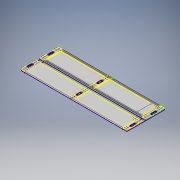
# Autodesk Inventor part: Fixture Base
Saved by Autodesk Inventor 2018 (Build 220112000, 112)
## iProperties
Created: 2016-04-07
Part Number: Fixture Base
Material: Generic
Document SubType Name: Modeling
Designer: Sam Clay
Density: 1 g/cm^3
Appearance: Default
Author: Sam Clay
Autodesk Inventor part; units mm, degrees
ref_plane "YZ Plane" through (0, 0, 0) normal (1, 0, 0) x (0, 1, 0)
ref_plane "XZ Plane" through (0, 0, 0) normal (0, 1, 0) x (-1, 0, 0)
ref_plane "XY Plane" through (0, 0, 0) normal (0, 0, 1) x (1, 0, 0)
sketch "Base Sketch" plane through (0, 0, 0) normal (0, 1, 0) x (-1, 0, 0)
  line L0 (0, 0) -> (1320.8, 0)
  line L1 (1320.8, 0) -> (1320.8, 254)
  line L2 (1320.8, 508) -> (0, 508)
  line L3 (0, 508) -> (0, 304.8)
  line L4 (0, 508) -> (-50.8, 508)
  line L5 (-50.8, 508) -> (-50.8, 304.8)
  line L6 (-50.8, 0) -> (0, 0)
  line L7 (0, 0) -> (0, 254)
  line L8 (1320.8, 508) -> (1371.6, 508)
  line L9 (1371.6, 508) -> (1371.6, 304.8)
  line L10 (1371.6, 0) -> (1320.8, 0)
  line L11 (1320.8, 0) -> (1320.8, 254)
  line L12 (1320.8, 254) -> (1320.8, 304.8)
  line L13 (1371.6, 254) -> (1371.6, 0)
  line L14 (0, 254) -> (0, 254)
  line L15 (-50.8, 254) -> (-50.8, 0)
  line L16 (1371.6, 254) -> (1320.8, 254)
  line L17 (1371.6, 304.8) -> (1320.8, 304.8)
  line L18 (1371.6, 304.8) -> (1371.6, 254)
  line L19 (1371.6, 254) -> (1371.6, 254)
  line L20 (1320.8, 254) -> (1320.8, 304.8)
  line L21 (1320.8, 304.8) -> (1320.8, 508)
  line L22 (0, 304.8) -> (0, 254)
  line L23 (0, 254) -> (0, 304.8)
  line L24 (-50.8, 254) -> (-50.8, 254)
  line L25 (-50.8, 304.8) -> (-50.8, 254)
  line L26 (1320.8, 254) -> (0, 254)
  line L27 (1320.8, 304.8) -> (0, 304.8)
  line L28 (0, 304.8) -> (-50.8, 304.8)
  line L29 (0, 254) -> (-50.8, 254)
  line L30 (0, 304.8) -> (0, 508)
  line L31 (0, 254) -> (0, 0)
  line L32 (1320.8, 254) -> (1320.8, 304.8)
  line L33 (1320.8, 304.8) -> (1320.8, 508)
  line L34 (1308.1, 0) -> (1308.1, 254)
  line L35 (12.7, 0) -> (12.7, 254)
  line L36 (1308.1, 304.8) -> (1308.1, 508) construction
  line L37 (12.7, 304.8) -> (12.7, 508) construction
  line L38 (1289.05, 323.85) -> (31.75, 323.85) construction
  line L39 (31.75, 323.85) -> (31.75, 488.95) construction
  line L40 (31.75, 488.95) -> (1289.05, 488.95) construction
  line L41 (1289.05, 488.95) -> (1289.05, 323.85) construction
  line L42 (660.4, 0) -> (660.4, 254)
  line L43 (660.4, 304.8) -> (660.4, 508)
  line L44 (711.2, 0) -> (711.2, 254)
  line L45 (711.2, 304.8) -> (711.2, 508)
  line L46 (647.7, 0) -> (647.7, 254)
  line L47 (647.7, 304.8) -> (647.7, 508) construction
  line L48 (628.65, 323.85) -> (628.65, 488.95) construction
  dimension "d89" = 17.78
  dimension "d0" = 1320.8
  dimension "d87" = 50.8
  dimension "d88" = 50.8
  dimension "d165" = 254
  dimension "d166" = 50.8
  dimension "d167" = 203.2
  dimension "d172" = 12.7
  dimension "d173" = 12.7
  dimension "d213" = 12.7
  dimension "d214" = 12.7
  dimension "d215" = 19.05
  dimension "d216" = 19.05
  dimension "d217" = 19.05
  dimension "d218" = 19.05
  dimension "d221" = 660.4
  dimension "d222" = 50.8
  dimension "d230" = 12.7
  dimension "d231" = 12.7
  dimension "d232" = 19.05
  constraints: 98 end point, 45 parallel, 40 perpendicular, 28 point on line, 14 coincident, 4 horizontal, 4 midpoint
  measures "d0" distance of L2.end L2.start
  measures "d87" distance of L6.end L6.start
  measures "d88" distance of L10.start L10.end
  measures "d165" distance between parallel lines of L16 L0
  measures "d166" distance between parallel lines of L16 L17
  measures "d167" distance between parallel lines of L2 L17
  measures "d172" distance between parallel lines of L34 L1
  measures "d173" distance between parallel lines of L31 L35
  measures "d213" distance between parallel lines of L33 L36
  measures "d214" distance between parallel lines of L3 L37
  measures "d215" distance between parallel lines of L38 L27
  measures "d216" distance between parallel lines of L36 L41
  measures "d217" distance between parallel lines of L37 L39
  measures "d218" distance between parallel lines of L2 L40
  measures "d221" distance between parallel lines of L42 L31
  measures "d222" distance between parallel lines of L44 L42
  measures "d230" distance between parallel lines of L46 L42
  measures "d231" distance between parallel lines of L47 L43
  measures "d232" distance between parallel lines of L48 L47
extrude "Lower Level" add sketch "Base Sketch" along normal blind 17.78 contours L6 L15 L29 L7 | L28 L5 L4 L3 | L21 L8 L9 L17 | L1 L16 L13 L10
extrude "Base" add sketch "Base Sketch" along normal blind 19.05 contours L7 L26 L35 L0 | L35 L26 L46 L0 | L46 L26 L42 L0 | L3 L2 L43 L27 | L42 L26 L44 L0 | L43 L2 L45 L27 | L44 L26 L34 L0 | L45 L2 L21 L27 | L34 L26 L1 L0
sketch "Tracks Sketch" plane through (0, 19.05, 0) normal (0, 1, 0) x (1, 0, 0)
  line L0 (-1320.8, 0) -> (-1320.8, -254) projected
  line L1 (0, -254) -> (0, 0) projected
  line L2 (-1320.8, -22.987) -> (0, -22.987)
  line L3 (-1320.8, -3.175) -> (0, -3.175)
  line L4 (-1320.8, -231.013) -> (0, -231.013)
  line L5 (-1320.8, -250.825) -> (0, -250.825)
  line L6 (-88.9, -40.767) -> (-1320.8, -40.767)
  line L7 (-1320.8, -40.767) -> (-1320.8, -231.013)
  line L8 (-88.9, -231.013) -> (-88.9, -40.767)
  circle A0 centre (-92.71, -44.577) radius 8.89
  line L9 (-1371.6, 0) -> (-1371.6, -254) projected
  line L10 (50.8, -508) -> (50.8, -304.8) projected
  line L11 (-1371.6, -508) -> (50.8, -508) projected
  line L12 (50.8, -304.8) -> (-1371.6, -304.8) projected
  line L13 (-1371.6, -254) -> (50.8, -254) projected
  line L14 (50.8, 0) -> (-1371.6, 0) projected
  line L15 (-1371.6, -304.8) -> (-1371.6, -508) projected
  line L16 (50.8, -254) -> (50.8, 0) projected
  point P0 (-660.4, -254)
  point P1 (-1320.8, -223.393)
  point P2 (-1422.4, -254)
  dimension "d170" = 19.812
  dimension "d171" = 19.812
  dimension "d174" = 88.9
  dimension "d175" = 17.78
  dimension "d178" = 17.78
  dimension "d179" = 5.08
  dimension "d180" = 5.08
  dimension "d219" = 3.175
  dimension "d220" = 3.175
  constraints: 14 end point, 6 point on line, 5 perpendicular, 1 centre point, 1 horizontal, 1 parallel, 6 other
  measures "d170" distance between parallel lines of L5 L4
  measures "d171" distance between parallel lines of L2 L3
  measures "d174" distance between parallel lines of L1 L8
  measures "d175" distance between parallel lines of L2 L6
  measures "d178" diameter of A0
  measures "d179" distance edge to line of A0 L6
  measures "d180" distance edge to line of A0 L8
  measures "d219" distance between parallel lines of L14 L3
  measures "d220" distance between parallel lines of L13 L5
extrude "Pocket side" cut sketch "Tracks Sketch" against normal blind 3.175 contours L6 A0 L8 L4 L0 | A0 L8 L6 | L6 L8 A0
extrude "Tracks" cut sketch "Tracks Sketch" against normal blind 11.43 contours L3 L1 L2 L0 | L4 L1 L5 L0
sketch "Handle Sketch" plane through (0, 17.78, 0) normal (0, 1, 0) x (1, 0, 0)
  line L0 (-1371.6, -254) -> (-1320.8, -254) projected
  line L1 (-1320.8, -40.767) -> (-1320.8, -22.987) projected
  line L2 (-1320.8, -22.987) -> (-1320.8, -3.175) projected
  line L3 (-1320.8, -250.825) -> (-1320.8, -40.767) projected
  line L4 (-1320.8, -254) -> (-1320.8, -250.825) projected
  line L5 (-1320.8, -3.175) -> (-1320.8, 0) projected
  line L6 (-1320.8, 0) -> (-1371.6, 0) projected
  line L7 (-1371.6, 0) -> (-1371.6, -254) projected
  line L8 (50.8, 0) -> (0, 0) projected
  line L9 (0, 0) -> (0, -3.175) projected
  line L10 (0, -3.175) -> (0, -22.987) projected
  line L11 (0, -22.987) -> (0, -231.013) projected
  line L12 (0, -231.013) -> (0, -250.825) projected
  line L13 (0, -250.825) -> (0, -254) projected
  line L14 (0, -254) -> (50.8, -254) projected
  line L15 (50.8, -254) -> (50.8, 0) projected
  line L16 (0, -508) -> (50.8, -508) projected
  line L17 (50.8, -508) -> (50.8, -304.8) projected
  line L18 (50.8, -304.8) -> (0, -304.8) projected
  line L19 (0, -304.8) -> (0, -508) projected
  line L20 (-1320.8, -508) -> (-1320.8, -304.8) projected
  line L21 (-1320.8, -304.8) -> (-1371.6, -304.8) projected
  line L22 (-1371.6, -304.8) -> (-1371.6, -508) projected
  line L23 (-1371.6, -508) -> (-1320.8, -508) projected
  line L24 (-1320.8, 0) -> (-1371.6, 0) construction
  line L25 (-1352.55, 0) -> (-1352.55, -508) construction
  line L26 (31.75, 0) -> (31.75, -508) construction
  line L27 (-1352.55, -88.9) -> (-1352.55, -165.1) construction
  line L28 (-1365.25, -101.6) -> (-1365.25, -152.4)
  line L29 (-1339.85, -152.4) -> (-1339.85, -101.6)
  arc A0 (-1339.85, -101.6) -> (-1365.25, -101.6) centre (-1352.55, -101.6) ccw
  arc A1 (-1365.25, -152.4) -> (-1339.85, -152.4) centre (-1352.55, -152.4) ccw
  line L30 (31.75, -88.9) -> (31.75, -165.1) construction
  line L31 (19.05, -101.6) -> (19.05, -152.4)
  line L32 (44.45, -152.4) -> (44.45, -101.6)
  arc A2 (44.45, -101.6) -> (19.05, -101.6) centre (31.75, -101.6) ccw
  arc A3 (19.05, -152.4) -> (44.45, -152.4) centre (31.75, -152.4) ccw
  line L33 (-1352.55, -368.3) -> (-1352.55, -444.5) construction
  line L34 (-1365.25, -381) -> (-1365.25, -431.8)
  line L35 (-1339.85, -431.8) -> (-1339.85, -381)
  arc A4 (-1339.85, -381) -> (-1365.25, -381) centre (-1352.55, -381) ccw
  arc A5 (-1365.25, -431.8) -> (-1339.85, -431.8) centre (-1352.55, -431.8) ccw
  line L36 (31.75, -368.3) -> (31.75, -444.5) construction
  line L37 (19.05, -381) -> (19.05, -431.8)
  line L38 (44.45, -431.8) -> (44.45, -381)
  arc A6 (44.45, -381) -> (19.05, -381) centre (31.75, -381) ccw
  arc A7 (19.05, -431.8) -> (44.45, -431.8) centre (31.75, -431.8) ccw
  arc A8 (-679.45, -381) -> (-704.85, -381) centre (-692.15, -381) ccw
  line L39 (-704.85, -381) -> (-704.85, -431.8)
  line L40 (-679.45, -431.8) -> (-679.45, -381)
  arc A9 (-704.85, -431.8) -> (-679.45, -431.8) centre (-692.15, -431.8) ccw
  arc A10 (-704.85, -152.4) -> (-679.45, -152.4) centre (-692.15, -152.4) ccw
  line L41 (-704.85, -101.6) -> (-704.85, -152.4)
  arc A11 (-679.45, -101.6) -> (-704.85, -101.6) centre (-692.15, -101.6) ccw
  line L42 (-679.45, -152.4) -> (-679.45, -101.6)
  point P0 (-1352.55, -25.4)
  point P1 (-1352.55, -50.8)
  point P2 (-1352.55, -203.2)
  point P3 (-1352.55, -228.6)
  point P4 (-1352.55, -317.5)
  point P5 (-1352.55, -342.9)
  point P6 (-1352.55, -469.9)
  point P7 (-1352.55, -495.3)
  point P8 (31.75, -495.3)
  point P9 (31.75, -469.9)
  point P10 (31.75, -342.9)
  point P11 (31.75, -317.5)
  point P12 (31.75, -228.6)
  point P13 (31.75, -203.2)
  point P14 (31.75, -50.8)
  point P15 (31.75, -25.4)
  point P16 (-1352.55, -127)
  point P17 (31.75, -127)
  point P18 (-1352.55, -406.4)
  point P19 (31.75, -406.4)
  point P20 (-692.15, -25.4)
  point P21 (-692.15, -50.8)
  point P22 (-692.15, -203.2)
  point P23 (-692.15, -228.6)
  point P24 (-692.15, -317.5)
  point P25 (-692.15, -342.9)
  point P26 (-692.15, -469.9)
  point P27 (-692.15, -495.3)
  dimension "d181" = 19.05
  dimension "d182" = 19.05
  dimension "d183" = 25.4
  dimension "d184" = 25.4
  dimension "d185" = 25.4
  dimension "d186" = 25.4
  dimension "d187" = 25.4
  dimension "d188" = 25.4
  dimension "d189" = 25.4
  dimension "d190" = 25.4
  dimension "d191" = 12.7
  dimension "d192" = 25.4
  dimension "d193" = 12.7
  dimension "d194" = 25.4
  dimension "d195" = 12.7
  dimension "d196" = 25.4
  dimension "d197" = 12.7
  dimension "d198" = 25.4
  dimension "d199" = 76.2
  dimension "d200" = 25.4
  dimension "d201" = 127
  dimension "d202" = 76.2
  dimension "d203" = 25.4
  dimension "d204" = 127
  dimension "d205" = 76.2
  dimension "d206" = 25.4
  dimension "d207" = 76.2
  dimension "d208" = 25.4
  dimension "d209" = 101.6
  dimension "d210" = 101.6
  dimension "d225" = 723.9
  constraints: 40 end point, 32 point on circle, 16 tangent, 12 centre point, 12 point on line, 4 midpoint, 4 parallel, 3 horizontal, 58 other
  measures "d183" distance from line of point (-1352.55, -25.4) L6
  measures "d184" distance of point (-1352.55, -25.4) point (-1352.55, -50.8)
  measures "d185" distance from line of L0 point (-1352.55, -228.6)
  measures "d186" distance of point (-1352.55, -203.2) point (-1352.55, -228.6)
  measures "d187" distance from line of point (31.75, -25.4) L8
  measures "d188" distance of point (31.75, -50.8) point (31.75, -25.4)
  measures "d189" distance from line of L14 point (31.75, -228.6)
  measures "d190" distance of point (31.75, -203.2) point (31.75, -228.6)
  measures "d191" distance from line of point (-1352.55, -317.5) L21
  measures "d192" distance of point (-1352.55, -342.9) point (-1352.55, -317.5)
  measures "d193" distance from line of L23 point (-1352.55, -495.3)
  measures "d194" distance of point (-1352.55, -469.9) point (-1352.55, -495.3)
  measures "d195" distance from line of L16 point (31.75, -495.3)
  measures "d196" distance of point (31.75, -469.9) point (31.75, -495.3)
  measures "d197" distance from line of point (31.75, -317.5) L18
  measures "d198" distance of point (31.75, -342.9) point (31.75, -317.5)
  measures "d199" distance of L27.start L27.end
  measures "d200" diameter of A1
  measures "d201" distance from line of L6 point (-1352.55, -127)
  measures "d202" distance of L30.start L30.end
  measures "d203" diameter of A3
  measures "d204" distance from line of L8 point (31.75, -127)
  measures "d205" distance of L33.start L33.end
  measures "d206" diameter of A5
  measures "d207" distance of L36.start L36.end
  measures "d208" diameter of A7
  measures "d209" distance from line of point (-1352.55, -406.4) L21
  measures "d210" distance from line of point (31.75, -406.4) L18
  measures "d225" distance of point (31.75, -25.4) point (-692.15, -25.4)
sketch "Origin Sketch" plane through (0, 19.05, 0) normal (0, 1, 0) x (1, 0, 0)
  line L0 (50.8, -254) -> (50.8, 0)
  line L1 (-1320.8, -40.767) -> (-100.7422, -40.767) projected
  line L2 (-12.7, 0) -> (-12.7, -254) projected
  line L3 (0, -304.8) -> (-1320.8, -304.8) projected
  line L4 (0, -304.8) -> (0, -508) projected
  line L5 (-1308.1, 0) -> (-1308.1, -254) projected
  line L6 (-711.2, 0) -> (-711.2, -254) projected
  line L7 (-660.4, 0) -> (-660.4, -254) projected
  line L8 (-647.7, 0) -> (-647.7, -254) projected
  line L9 (-711.2, -304.8) -> (-711.2, -508) projected
  line L10 (-660.4, -304.8) -> (-660.4, -508) projected
  line L11 (-647.7, -304.8) -> (-647.7, -508) construction
  line L12 (-628.65, -323.85) -> (-628.65, -488.95) construction
  line L13 (-1289.05, -323.85) -> (-31.75, -323.85) construction
  line L14 (-31.75, -488.95) -> (-1289.05, -488.95) construction
  line L15 (-1289.05, -488.95) -> (-1289.05, -323.85) construction
  line L16 (-1308.1, -304.8) -> (-1308.1, -508) construction
  line L17 (-31.75, -323.85) -> (-31.75, -488.95) construction
  line L18 (-12.7, -304.8) -> (-12.7, -508) construction
  point P0 (0, 0)
  point P1 (-12.7, -40.767)
  point P2 (-711.2, -508)
  point P3 (50.8, -508)
  point P4 (-25.4, -317.5)
  dimension "d211" = 12.7
  dimension "d212" = 25.4
  constraints: 2 end point, 2 point on line
  measures "d211" distance from line of L3 point (-25.4, -317.5)
  measures "d212" distance from line of L4 point (-25.4, -317.5)
extrude "Handles" cut sketch "Handle Sketch" along normal through all both and the other way through all contours A0 L29 A1 L28 | A2 L32 A3 L31 | A4 L35 A5 L34 | A6 L38 A7 L37 | L40 A9 L39 A8 | L41 A11 L42 A10
body "Solid1"
